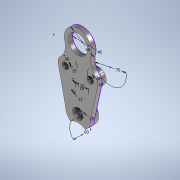
# Autodesk Inventor part: Деталь1
Saved by Autodesk Inventor 2020 (Build 240168000, 168)
## iProperties
Created: 2020-03-15
Part Number: Деталь1
Material: Сталь, гальванизированная
Document SubType Name: Modeling
Designer: User
Density: 7.85 g/cm^3
Appearance: Гальванизированная
Author: User
Autodesk Inventor part; units mm, degrees
ref_plane "YZ Plane" through (0, 0, 0) normal (1, 0, 0) x (0, 1, 0)
ref_plane "XZ Plane" through (0, 0, 0) normal (0, 1, 0) x (-1, 0, 0)
ref_plane "XY Plane" through (0, 0, 0) normal (0, 0, 1) x (1, 0, 0)
sketch "Эскиз1" plane through (0, 0, 0) normal (0, 0, 1) x (1, 0, 0)
  circle A0 centre (0, 0) radius 33
  circle A1 centre (-30, -60) radius 7.5
  circle A2 centre (30, -60) radius 7.5
  arc A3 (42.6567, -72.7987) -> (17.0554, -47.4925) centre (30, -60) ccw
  arc A4 (-17.0554, -47.4925) -> (-42.6567, -72.7987) centre (-30, -60) ccw
  circle A5 centre (0, -145) radius 12.5
  arc A6 (32.1885, -7.2731) -> (42.7278, -47.2719) centre (68.2848, -19.1501) ccw
  arc A7 (-17.8315, -46.7362) -> (17.8315, -46.7362) centre (0, -29.2137) ccw
  arc A8 (-42.7278, -47.2719) -> (-32.1885, -7.2731) centre (-68.2848, -19.1501) ccw
  line L0 (-15, -102.5) -> (-15, -116.1893)
  line L1 (15, -102.5) -> (15, -116.1893)
  line L2 (-15, -102.5) -> (-15, -92.1226)
  line L3 (15, -102.5) -> (15, -92.1226)
  arc A9 (-15, -92.7535) -> (-18.8083, -87.5797) centre (-19.99, -92.4381) ccw
  arc A10 (-43.0534, -72.3939) -> (-18.1041, -87.8074) centre (0, -30.6039) ccw
  arc A11 (18.1041, -87.8074) -> (43.0534, -72.3939) centre (0, -30.6039) ccw
  arc A12 (-17.6847, -120.7667) -> (-15, -115.3217) centre (-20.9843, -115.7555) ccw
  arc A13 (18.8083, -87.5797) -> (15, -92.7535) centre (19.99, -92.4381) ccw
  arc A14 (15, -115.3217) -> (17.6847, -120.7667) centre (20.9843, -115.7555) ccw
  arc A15 (17.6618, -169.25) -> (-17.6618, -169.25) centre (0, -193.5) ccw
  arc A16 (-17.2936, -120.4861) -> (-17.6618, -169.25) centre (0, -145) ccw
  arc A17 (17.6618, -169.25) -> (17.2936, -120.4861) centre (0, -145) ccw
  line L4 (29.9991, -144.7735) -> (47.5895, -63.8221)
  line L5 (-29.9991, -144.7735) -> (-47.5895, -63.8221)
  circle A18 centre (0, 0) radius 23
  point P0 (41.8771, -46.4746)
  point P1 (31.2765, -10.5253)
  point P2 (-31.2765, -10.5253)
  point P3 (-41.8771, -46.4746)
  point P4 (15, -92.7535)
  dimension "d1" = 66
  dimension "d5" = 15
  dimension "d6" = 15
  dimension "d7" = 36
  dimension "d8" = 36
  dimension "d10" = 25
  dimension "d13" = 76
  dimension "d17" = 30
  dimension "d18" = 10
  dimension "d19" = 12
  dimension "d22" = 60
  dimension "d30" = 46
  constraints: 49 point on circle, 18 centre point, 12 end point, 4 coincident, 2 point on line, 2 vertical, 1 tangent, 3 other
  measures "d5" diameter of A1
  measures "d6" diameter of A2
  measures "d7" diameter of A3
  measures "d8" diameter of A4
  measures "d10" diameter of A5
  measures "d13" diameter of A6
  measures "d17" distance of L1.start L0.start
  measures "d18" diameter of A9
  measures "d19" diameter of A12
  measures "d22" diameter of A15
  measures "d30" diameter of A18
sketch "Эскиз2" plane through (0, 0, 0) normal (0, 0, 1) x (1, 0, 0)
  point P0 (0, 0)
extrude "Выдавливание1" add sketch "Эскиз1" along normal blind 10 contours A0 A6 A8 | A8 A0 | A0 A6 | A0 A6 A3 A7 A4 A8 | A8 A4 | A4 A7 A3 A6 A11 A13 L3 L1 A14 A17 A15 A16 A12 L0 L2 A9 A10 A8 | A3 A6 | A4 A7 | A7 A3 | A4 A10 A9 L2 L0 A12 A16 L5 | L4 A17 A14 L1 L3 A13 A11 A3 | A16 A12 | A14 A17 | A9 A10 | A11 A13 | L0 A12 | A14 L1 | A9 L2 | L3 A13 | A1 | A2 | A5 | A18
extrude "Выдавливание2" add sketch "Эскиз1" against normal blind 10 contours A4 A7 A3 A6 A11 A13 L3 L1 A14 A17 A15 A16 A12 L0 L2 A9 A10 A8
extrude "Выдавливание3" cut sketch "Эскиз1" along normal blind 10 contours A5
extrude "Выдавливание4" cut sketch "Эскиз1" along normal blind 10 contours A2
extrude "Выдавливание5" cut sketch "Эскиз1" along normal blind 10 contours A1
extrude "Выдавливание6" cut sketch "Эскиз1" along normal blind 10 contours A18
